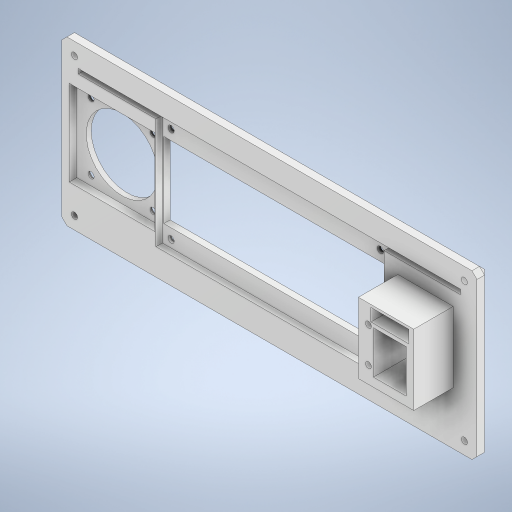
# Autodesk Inventor part: face_frontale
Saved by Autodesk Inventor 2024.2 (Build 282272000, 272)
## iProperties
Created: 2024-05-07
Part Number: face_frontale
Material: PVC, non plastifié
Document SubType Name: Modeling
Designer: michgae
Density: 1.29 g/cm^3
Appearance: Lisse - Blanc
Author: michgae
Autodesk Inventor part; units mm, degrees
ref_plane "YZ Plane" through (0, 0, 0) normal (1, 0, 0) x (0, 1, 0)
ref_plane "XZ Plane" through (0, 0, 0) normal (0, 1, 0) x (-1, 0, 0)
ref_plane "XY Plane" through (0, 0, 0) normal (0, 0, 1) x (1, 0, 0)
sketch "Esquisse1" plane through (0, 0, 0) normal (0, 0, 1) x (1, 0, 0)
  line L0 (-82.5, -32.5) -> (82.5, -32.5)
  line L1 (82.5, -32.5) -> (82.5, 32.5)
  line L2 (82.5, 32.5) -> (-82.5, 32.5)
  line L3 (-82.5, 32.5) -> (-82.5, -32.5)
  line L4 (-115.5, 0) -> (115.5, 0) projected
  line L5 (0, -45.5) -> (0, 45.5) projected
  line L6 (-44.5, 15) -> (44.5, 15)
  line L7 (44.5, 15) -> (44.5, -15)
  line L8 (44.5, -15) -> (-44.5, -15)
  line L9 (-44.5, -15) -> (-44.5, 15)
  line L10 (-44.6, 22) -> (44.6, 22)
  line L11 (44.6, 22) -> (44.6, -22)
  line L12 (44.6, -22) -> (-44.6, -22)
  line L13 (-44.6, -22) -> (-44.6, 22)
  circle A0 centre (-41.6, 19) radius 1.3
  circle A1 centre (41.6, 19) radius 1.3
  circle A2 centre (-41.6, -19) radius 1.3
  circle A3 centre (41.6, -19) radius 1.3
  line L14 (-45.6, -17) -> (-79.6, -17)
  line L15 (-79.6, -17) -> (-79.6, 17)
  line L16 (-79.6, 17) -> (-45.6, 17)
  line L17 (-45.6, 17) -> (-45.6, -17)
  circle A4 centre (-49.3, -13.3) radius 1.25
  circle A5 centre (-49.3, 13.3) radius 1.25
  circle A6 centre (-73.9, -13.3) radius 1.25
  circle A7 centre (-73.9, 13.3) radius 1.25
  circle A8 centre (-61.6, 0) radius 14.25
  circle A9 centre (-77.5, -27.5) radius 1.25
  circle A10 centre (77.5, -27.5) radius 1.25
  circle A11 centre (-77.5, 27.5) radius 1.25
  circle A12 centre (77.5, 27.5) radius 1.25
  circle A13 centre (63.55, 0) radius 4
  line L18 (-76, 23.9) -> (76, 23.9)
  line L19 (76, 23.9) -> (76, 22)
  line L20 (76, 22) -> (-76, 22)
  line L21 (-76, 22) -> (-76, 23.9)
  line L22 (82.5, 32.5) -> (-82.5, 32.5)
  line L23 (-82.5, 32.5) -> (-82.5, 30.5)
  line L24 (-82.5, 30.5) -> (82.5, 30.5)
  line L25 (82.5, 30.5) -> (82.5, 32.5)
  line L26 (-44.6, -22) -> (-45.1, -22)
  line L27 (-45.1, -22) -> (-45.1, 22)
  line L28 (-45.1, 22) -> (-44.6, 22)
  line L29 (-44.6, 22) -> (-44.6, -22)
  line L30 (44.6, -22) -> (45.6, -22)
  line L31 (45.6, -22) -> (45.6, 22)
  line L32 (45.6, 22) -> (44.6, 22)
  line L33 (44.6, 22) -> (44.6, -22)
  point P0 (0, 0)
  point P1 (82.5, 30.5)
  point P2 (-44.6, 0)
  point P3 (-45.1, 0)
  dimension "d0" = 165
  dimension "d1" = 65
  dimension "d2" = 30
  dimension "d3" = 89
  dimension "d4" = 89.2
  dimension "d6" = 2.6
  dimension "d31" = 34
  dimension "d32" = 34
  dimension "d33" = 1
  dimension "d34" = 2.5
  dimension "d35" = 3.7
  dimension "d36" = 3.7
  dimension "d39" = 24.6
  dimension "d44" = 28.5
  dimension "d45" = 16
  dimension "d53" = 2.5
  dimension "d54" = 5
  dimension "d55" = 5
  dimension "d58" = 155
  dimension "d68" = 8
  dimension "d116" = 44.6
  dimension "d119" = 63.55
  dimension "d122" = 22
  dimension "d124" = 44.6
  dimension "d125" = 22
  dimension "d127" = 152
  dimension "d128" = 1.9
  dimension "d131" = 2
  dimension "d134" = 41.6
  dimension "d135" = 19
  dimension "d136" = 82.5
  dimension "d137" = 30.5
  dimension "d138" = 44.6
  dimension "d139" = 22
  dimension "d140" = 41.6
  dimension "d141" = 44.6
  dimension "d142" = 22
  dimension "d143" = 0.5
  dimension "d144" = 1
  constraints: 64 end point, 16 parallel, 14 centre point, 10 horizontal, 8 perpendicular, 6 symmetric about line, 5 point on line, 1 collinear, 20 other
  measures "d0" distance of L0.start L0.end
  measures "d1" distance of L0.end L1.end
  measures "d2" distance of L6.end L7.end
  measures "d3" distance of L6.start L6.end
  measures "d4" distance of L10.end L10.start
  measures "d6" diameter of A0
  measures "d31" distance of L15.end L16.end
  measures "d32" distance of L14.end L15.end
  measures "d33" distance between parallel lines of L13 L17
  measures "d34" diameter of A4
  measures "d35" distance from line of L14 A4.centre
  measures "d36" distance from line of L17 A4.centre
  measures "d39" distance of A4.centre A6.centre
  measures "d44" diameter of A8
  measures "d45" distance from line of L17 A8.centre
  measures "d53" diameter of A9
  measures "d54" distance from line of L0 A9.centre
  measures "d55" distance from line of L3 A9.centre
  measures "d58" distance of A9.centre A10.centre
  measures "d68" diameter of A13
  measures "d116" distance between parallel lines of L11 L5
  measures "d119" distance from line of A13.centre L5
  measures "d122" distance between parallel lines of L12 L4
  measures "d124" distance from line of point (44.6, 22) L5
  measures "d125" distance from line of point (44.6, 22) L4
  measures "d127" distance of L19.end L20.end
  measures "d128" distance of L20.end L18.start
  measures "d131" distance of L23.end L22.end
  measures "d134" distance from line of L5 A0.centre
  measures "d135" distance from line of L4 A0.centre
  measures "d136" distance from line of point (82.5, 30.5) L5
  measures "d137" distance from line of point (82.5, 30.5) L4
  measures "d138" distance from line of point (44.6, 22) L5
  measures "d139" distance from line of point (44.6, 22) L4
  measures "d140" distance from line of A1.centre L5
  measures "d141" distance from line of point (-44.6, 22) L5
  measures "d142" distance from line of point (-44.6, 22) L4
  measures "d143" distance of L27.end L28.end
  measures "d144" distance of L32.end L31.end
extrude "Extrusion1" add sketch "Esquisse1" against normal blind 5 contours L3 L4 L15 L14 L17 L27 L26 L12 L5 L0 | L5 L12 L30 L31 L4 A13 L1 L0 | L3 L24 L5 L18 L21 L20 L27 L4 L17 L16 L15 | L12 L13 L4 L9 L8 L5 | L5 L8 L7 L4 L11 L12 | L3 L2 L5 L24 | L15 L16 L17 L4 A8 | L4 A8 L17 L14 L15 | L4 A13 L31 L20 L19 L18 L5 L24 L1 | L11 L4 L31 L30 | L26 L27 L4 L13 | L5 L2 L1 L24 | A8 L4 | L4 A8 | A13 L4 | L4 A13 | L11 L20 L31 L4 | L4 L7 L6 L5 L10 L11 | L13 L10 L5 L6 L9 L4 | L4 L27 L20 L13 | L18 L19 L20 L10 L5 | L5 L10 L20 L21 L18 | A4 | A5 | A6 | A7 | A9 | A10 | A11 | A12
extrude "Extrusion2" cut sketch "Esquisse1" against normal blind 2.5 contours L12 L13 L4 L9 L8 L5 | L5 L8 L7 L4 L11 L12 | L8 L9 L4 L5 | L5 L4 L7 L8 | L11 L4 L31 L30 | L26 L27 L4 L13 | L5 L6 L7 L4 | L4 L9 L6 L5 | L11 L20 L31 L4 | L4 L7 L6 L5 L10 L11 | L13 L10 L5 L6 L9 L4 | L4 L27 L20 L13
chamfer "Chanfrein1" distance 1.5 angle 45 4 edges at (40.3, 19, -5) (-42.9, 19, -5) (40.3, -19, -5) (-42.9, -19, -5)
extrude "Extrusion3" cut sketch "Esquisse1" against normal through all contours A8 L4 | L4 A8 | A4 | A5 | A6 | A7
extrude "Extrusion4" cut sketch "Esquisse1" against normal blind 3 contours L15 L16 L17 L4 A8 | L4 A8 L17 L14 L15
chamfer "Chanfrein2" distance 1.5 angle 45 4 edges at (-75.15, 13.3, -5) (-50.55, -13.3, -5) (-75.15, -13.3, -5) (-50.55, 13.3, -5)
extrude "Extrusion5" cut sketch "Esquisse1" against normal through all contours A9 | A10 | A11 | A12
chamfer "Chanfrein3" distance 1.5 angle 45 4 edges at (-78.75, -27.5, -5) (-78.75, 27.5, -5) (76.25, -27.5, -5) (76.25, 27.5, -5)
extrude "Extrusion6" cut sketch "Esquisse1" against normal through all contours A13 L4 | L4 A13
sketch "Esquisse3" plane through (0, 0, 0) normal (0, 0, 1) x (1, 0, 0)
  line L0 (70.05, -8) -> (57.05, -8)
  line L1 (57.05, -8) -> (57.05, 9)
  line L2 (57.05, 9) -> (70.05, 9)
  line L3 (70.05, 9) -> (70.05, -8)
  circle A0 centre (63.55, 0) radius 4 projected
  line L4 (-115.5, 0) -> (115.5, 0) projected
  line L5 (73.05, -11.5) -> (51.05, -11.5)
  line L6 (51.05, -11.5) -> (51.05, 16.5)
  line L7 (51.05, 16.5) -> (73.05, 16.5)
  line L8 (73.05, 16.5) -> (73.05, -11.5)
  line L9 (63.55, -11.5) -> (63.55, 16.9619)
  circle A1 centre (55.05, -4.85) radius 1.2
  circle A2 centre (55.05, 9.07) radius 1.2
  point P0 (0, 0)
  dimension "d77" = 13
  dimension "d78" = 17
  dimension "d79" = 6.5
  dimension "d80" = 11.5
  dimension "d83" = 22
  dimension "d84" = 28
  dimension "d86" = 8
  dimension "d97" = 6
  dimension "d98" = 2.4
  dimension "d99" = 9.5
  dimension "d100" = 16.9619
  dimension "d101" = 9.07
  dimension "d102" = 4.85
  dimension "d103" = 18
  dimension "d104" = 18
  constraints: 18 end point, 4 parallel, 3 perpendicular, 2 centre point, 1 equal radius, 1 horizontal, 1 point on line
  measures "d77" distance of L1.end L2.end
  measures "d78" distance of L0.end L1.end
  measures "d79" distance from line of A0.centre L3
  measures "d80" distance from line of L5 A0.centre
  measures "d83" distance of L5.start L5.end
  measures "d84" distance of L7.end L5.start
  measures "d86" distance between parallel lines of L0 L4
  measures "d97" distance between parallel lines of L6 L1
  measures "d98" diameter of A2
  measures "d99" distance between parallel lines of L9 L8
  measures "d100" distance from line of L9.end L4
  measures "d101" distance from line of A2.centre L4
  measures "d102" distance from line of A1.centre L4
  measures "d103" distance from line of A2.centre L8
  measures "d104" distance from line of A1.centre L8
extrude "Extrusion7" add sketch "Esquisse3" along normal blind 15.686 contours L3 L4 L8 L5 L9 L0 | L9 L5 L6 L4 L1 L0 | L3 L2 L9 L7 L8 L4 | L4 L6 L7 L9 L2 L1
sketch "Esquisse4" plane through (0, 0, 15.686) normal (0, 0, 1) x (1, 0, 0)
  line L0 (71.05, 15.5) -> (56.05, 15.5)
  line L1 (56.05, 15.5) -> (56.05, 10.5)
  line L2 (56.05, 10.5) -> (71.05, 10.5)
  line L3 (71.05, 10.5) -> (71.05, 15.5)
  line L4 (73.05, -11.5) -> (73.05, 16.5) projected
  line L5 (73.05, 16.5) -> (51.05, 16.5) projected
  line L6 (51.05, 16.5) -> (51.05, -11.5) projected
  point P0 (0, 0)
  dimension "d106" = 2
  dimension "d107" = 1
  dimension "d108" = 5
  dimension "d109" = 5
  constraints: 8 end point, 2 parallel, 1 horizontal, 1 perpendicular
  measures "d106" distance between parallel lines of L4 L3
  measures "d107" distance between parallel lines of L5 L0
  measures "d108" distance between parallel lines of L6 L1
  measures "d109" distance of L0.end L1.end
extrude "Extrusion8" cut sketch "Esquisse4" against normal blind 5
extrude "Extrusion10" cut sketch "Esquisse1" against normal blind 2.5 contours L18 L19 L20 L10 L5 | L5 L10 L20 L21 L18
chamfer "Chanfrein4" distance 2 angle 45 8 edges at (0, -32.5, -5) (82.5, 0, -5) (0, 32.5, -5) (-82.5, 0, -5) (82.5, -32.5, -2.5) (82.5, 32.5, -2.5) (-82.5, 32.5, -2.5) (-82.5, -32.5, -2.5)
